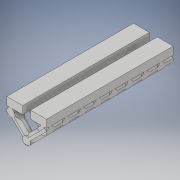
# Autodesk Inventor part: Basic_rail
Saved by Autodesk Inventor 2018.2 (Build 222227000, 227)
## iProperties
Created: 2018-04-02
Part Number: Basic_rail
Material: Generic
Document SubType Name: Modeling
Designer: martin
Density: 1 g/cm^3
Appearance: Default
Author: martin
Autodesk Inventor part; units mm, degrees
ref_plane "YZ Plane" through (0, 0, 0) normal (1, 0, 0) x (0, 1, 0)
ref_plane "XZ Plane" through (0, 0, 0) normal (0, 1, 0) x (-1, 0, 0)
ref_plane "XY Plane" through (0, 0, 0) normal (0, 0, 1) x (1, 0, 0)
sketch "Sketch1" plane through (0, 0, 0) normal (0, 0, 1) x (1, 0, 0)
  line L0 (0.0508, 0.0012) -> (1.1089, 0.0012)
  line L1 (1.1089, 0.0012) -> (2.1671, 1.0594)
  line L2 (2.1671, 1.0594) -> (2.1671, 2.1175)
  line L3 (2.1671, 2.1175) -> (1.1084, 3.1762)
  line L4 (1.1084, 3.1762) -> (0.0503, 3.1762)
  line L5 (0.0503, 3.1762) -> (-1.0079, 2.118)
  line L6 (-1.0079, 2.118) -> (-1.0079, 1.0599)
  line L7 (-1.0079, 1.0599) -> (0.0508, 0.0012)
  line L8 (6.4008, 0.0012) -> (7.4589, 0.0012)
  line L9 (7.4589, 0.0012) -> (8.5171, 1.0594)
  line L10 (8.5171, 1.0594) -> (8.5171, 2.1175)
  line L11 (8.5171, 2.1175) -> (7.4584, 3.1762)
  line L12 (7.4584, 3.1762) -> (6.4003, 3.1762)
  line L13 (6.4003, 3.1762) -> (5.3421, 2.118)
  line L14 (5.3421, 2.118) -> (5.3421, 1.0599)
  line L15 (5.3421, 1.0599) -> (6.4008, 0.0012)
  line L16 (0.0508, 0.0012) -> (1.1089, 0.0012)
  line L17 (1.1089, 0.0012) -> (2.1671, 1.0594)
  line L18 (2.1671, 1.0594) -> (2.1671, 2.1175)
  line L19 (2.1671, 2.1175) -> (1.1084, 3.1762)
  line L20 (1.1084, 3.1762) -> (0.0503, 3.1762)
  line L21 (0.0503, 3.1762) -> (-1.0079, 2.118)
  line L22 (-1.0079, 2.118) -> (-1.0079, 1.0599)
  line L23 (-1.0079, 1.0599) -> (0.0508, 0.0012)
  line L24 (12.7508, 0.0012) -> (13.8089, 0.0012)
  line L25 (13.8089, 0.0012) -> (14.8671, 1.0594)
  line L26 (14.8671, 1.0594) -> (14.8671, 2.1175)
  line L27 (14.8671, 2.1175) -> (13.8084, 3.1762)
  line L28 (13.8084, 3.1762) -> (12.7503, 3.1762)
  line L29 (12.7503, 3.1762) -> (11.6921, 2.118)
  line L30 (11.6921, 2.118) -> (11.6921, 1.0599)
  line L31 (11.6921, 1.0599) -> (12.7508, 0.0012)
  point P0 (0, 0)
  dimension "d0" = 0.0508
  dimension "d1" = 1.109
  dimension "d2" = 1.0582
  dimension "d3" = 135
  dimension "d4" = 135
  dimension "d5" = 135
  dimension "d6" = 3.175
  dimension "d8" = 1.0582
  dimension "d9" = 135
  dimension "d10" = 1.0582
  dimension "d11" = 1.0582
  dimension "d12" = 1.0582
  dimension "d13" = 135
  dimension "d14" = 135
  dimension "d15" = 135
  dimension "d16" = 3.175
  dimension "d17" = 3.175
  dimension "d18" = 1.0582
  dimension "d19" = 135
  dimension "d20" = 1.0582
  dimension "d21" = 1.0582
  dimension "d22" = 1.0582
  dimension "d23" = 135
  dimension "d24" = 135
  dimension "d25" = 135
  dimension "d26" = 3.175
  dimension "d27" = 3.175
  dimension "d28" = 1.0582
  dimension "d29" = 135
  dimension "d30" = 1.0582
  dimension "d31" = 1.0582
  dimension "d32" = 1.0582
  dimension "d33" = 135
  dimension "d34" = 135
  dimension "d35" = 135
  dimension "d36" = 3.175
  dimension "d37" = 3.175
  dimension "d38" = 1.0582
  dimension "d39" = 135
  dimension "d40" = 1.0582
  dimension "d41" = 1.0582
  dimension "d52" = 3.175
  dimension "d54" = 3.175
  constraints: 64 end point, 12 parallel, 4 horizontal, 4 perpendicular
  measures "d0" distance of point (0, 0) L0.start
  measures "d1" distance of L0.end point (0, 0)
  measures "d2" horizontal distance of L0.end L1.end
  measures "d3" angle of L0 L1
  measures "d4" angle of L2 L1
  measures "d5" angle of L3 L2
  measures "d6" distance between parallel lines of L0 L4
  measures "d8" distance of L0.start L0.end
  measures "d9" angle of L0 L7
  measures "d10" distance of L5.end L6.end
  measures "d11" distance of L3.end L4.end
  measures "d12" horizontal distance of L8.end L9.end
  measures "d13" angle of L8 L9
  measures "d14" angle of L10 L9
  measures "d15" angle of L11 L10
  measures "d16" distance between parallel lines of L8 L12
  measures "d17" distance between parallel lines of L14 L10
  measures "d18" distance of L8.start L8.end
  measures "d19" angle of L8 L15
  measures "d20" distance of L13.end L14.end
  measures "d21" distance of L11.end L12.end
  measures "d22" horizontal distance of L16.end L17.end
  measures "d23" angle of L16 L17
  measures "d24" angle of L18 L17
  measures "d25" angle of L19 L18
  measures "d26" distance between parallel lines of L16 L20
  measures "d27" distance between parallel lines of L22 L18
  measures "d28" distance of L16.start L16.end
  measures "d29" angle of L16 L23
  measures "d30" distance of L21.end L22.end
  measures "d31" distance of L19.end L20.end
  measures "d32" horizontal distance of L24.end L25.end
  measures "d33" angle of L24 L25
  measures "d34" angle of L26 L25
  measures "d35" angle of L27 L26
  measures "d36" distance between parallel lines of L24 L28
  measures "d37" distance between parallel lines of L30 L26
  measures "d38" distance of L24.start L24.end
  measures "d39" angle of L24 L31
  measures "d40" distance of L29.end L30.end
  measures "d41" distance of L27.end L28.end
  measures "d52" distance between parallel lines of L14 L18
  measures "d54" distance between parallel lines of L30 L10
extrude "Extrusion1" add sketch "Sketch1" along normal mid plane 50.8
sketch "Sketch2" plane through (14.8671, 1.0594, 25.4) normal (1, 0, 0) x (0, 0, -1)
  line L0 (1.0587, -1.0587) -> (2.1168, -1.0587)
  line L1 (2.1168, -1.0587) -> (3.175, -0.0005)
  line L2 (3.175, -0.0005) -> (3.175, 1.0577)
  line L3 (3.175, 1.0577) -> (2.1163, 2.1163)
  line L4 (2.1163, 2.1163) -> (1.0582, 2.1163)
  line L5 (1.0582, 2.1163) -> (0, 1.0582)
  line L6 (0, 1.0582) -> (0, 0)
  line L7 (0, 0) -> (1.0587, -1.0587)
  line L8 (7.4087, -1.0587) -> (8.4668, -1.0587)
  line L9 (8.4668, -1.0587) -> (9.525, -0.0005)
  line L10 (9.525, -0.0005) -> (9.525, 1.0577)
  line L11 (9.525, 1.0577) -> (8.4663, 2.1163)
  line L12 (8.4663, 2.1163) -> (7.4082, 2.1163)
  line L13 (7.4082, 2.1163) -> (6.35, 1.0582)
  line L14 (6.35, 1.0582) -> (6.35, 0)
  line L15 (6.35, 0) -> (7.4087, -1.0587)
  line L16 (1.0587, -1.0587) -> (2.1168, -1.0587)
  line L17 (2.1168, -1.0587) -> (3.175, -0.0005)
  line L18 (3.175, -0.0005) -> (3.175, 1.0577)
  line L19 (3.175, 1.0577) -> (2.1163, 2.1163)
  line L20 (2.1163, 2.1163) -> (1.0582, 2.1163)
  line L21 (1.0582, 2.1163) -> (0, 1.0582)
  line L22 (0, 1.0582) -> (0, 0)
  line L23 (0, 0) -> (1.0587, -1.0587)
  line L24 (13.7587, -1.0587) -> (14.8168, -1.0587)
  line L25 (14.8168, -1.0587) -> (15.875, -0.0005)
  line L26 (15.875, -0.0005) -> (15.875, 1.0577)
  line L27 (15.875, 1.0577) -> (14.8163, 2.1163)
  line L28 (14.8163, 2.1163) -> (13.7582, 2.1163)
  line L29 (13.7582, 2.1163) -> (12.7, 1.0582)
  line L30 (12.7, 1.0582) -> (12.7, 0)
  line L31 (12.7, 0) -> (13.7587, -1.0587)
  line L32 (21.1182, 2.1163) -> (20.06, 2.1163)
  line L33 (21.1663, 2.1163) -> (20.1082, 2.1163)
  line L34 (20.1082, 2.1163) -> (19.05, 1.0582)
  line L35 (20.06, 2.1163) -> (19.0018, 1.0582)
  line L36 (22.225, 1.0577) -> (21.1663, 2.1163)
  line L37 (22.1768, 1.0577) -> (21.1182, 2.1163)
  line L38 (19.05, 1.0582) -> (19.05, 0)
  line L39 (19.0018, 1.0582) -> (19.0018, 0)
  line L40 (22.225, -0.0005) -> (22.225, 1.0577)
  line L41 (22.1768, -0.0005) -> (22.1768, 1.0577)
  line L42 (20.1087, -1.0587) -> (21.1668, -1.0587)
  line L43 (20.0605, -1.0587) -> (21.1187, -1.0587)
  line L44 (19.0018, 0) -> (20.0605, -1.0587)
  line L45 (19.05, 0) -> (20.1087, -1.0587)
  line L46 (21.1187, -1.0587) -> (22.1768, -0.0005)
  line L47 (21.1668, -1.0587) -> (22.225, -0.0005)
  line L48 (31.7018, 1.0582) -> (31.7018, 0)
  line L49 (32.76, 2.1163) -> (31.7018, 1.0582)
  line L50 (31.7018, 0) -> (32.7605, -1.0587)
  line L51 (33.8182, 2.1163) -> (32.76, 2.1163)
  line L52 (32.7605, -1.0587) -> (33.8187, -1.0587)
  line L53 (33.8187, -1.0587) -> (34.8768, -0.0005)
  line L54 (34.8768, -0.0005) -> (34.8768, 1.0577)
  line L55 (34.8768, 1.0577) -> (33.8182, 2.1163)
  line L56 (25.3518, 1.0582) -> (25.3518, 0)
  line L57 (26.41, 2.1163) -> (25.3518, 1.0582)
  line L58 (25.3518, 0) -> (26.4105, -1.0587)
  line L59 (27.4682, 2.1163) -> (26.41, 2.1163)
  line L60 (26.4105, -1.0587) -> (27.4687, -1.0587)
  line L61 (27.4687, -1.0587) -> (28.5268, -0.0005)
  line L62 (28.5268, -0.0005) -> (28.5268, 1.0577)
  line L63 (28.5268, 1.0577) -> (27.4682, 2.1163)
  line L64 (38.0518, 1.0582) -> (38.0518, 0)
  line L65 (38.0518, 0) -> (39.1105, -1.0587)
  line L66 (39.11, 2.1163) -> (38.0518, 1.0582)
  line L67 (39.1105, -1.0587) -> (40.1687, -1.0587)
  line L68 (40.1682, 2.1163) -> (39.11, 2.1163)
  line L69 (40.1687, -1.0587) -> (41.2268, -0.0005)
  line L70 (41.2268, 1.0577) -> (40.1682, 2.1163)
  line L71 (41.2268, -0.0005) -> (41.2268, 1.0577)
  line L72 (44.4018, 1.0582) -> (44.4018, 0)
  line L73 (44.4018, 0) -> (45.4605, -1.0587)
  line L74 (45.46, 2.1163) -> (44.4018, 1.0582)
  line L75 (45.4605, -1.0587) -> (46.5187, -1.0587)
  line L76 (46.5182, 2.1163) -> (45.46, 2.1163)
  line L77 (46.5187, -1.0587) -> (47.5768, -0.0005)
  line L78 (47.5768, -0.0005) -> (47.5768, 1.0577)
  line L79 (47.5768, 1.0577) -> (46.5182, 2.1163)
  point P0 (25.4, -1.0594)
  point P1 (1.0079, -1.0599)
  point P2 (20.0579, -1.0599)
  dimension "d57" = 0.0508
  dimension "d58" = 1.109
  dimension "d59" = 1.0582
  dimension "d60" = 135
  dimension "d61" = 135
  dimension "d62" = 135
  dimension "d63" = 3.175
  dimension "d64" = 1.0582
  dimension "d65" = 135
  dimension "d66" = 1.0582
  dimension "d67" = 1.0582
  dimension "d68" = 1.0582
  dimension "d69" = 135
  dimension "d70" = 135
  dimension "d71" = 135
  dimension "d72" = 3.175
  dimension "d73" = 3.175
  dimension "d74" = 1.0582
  dimension "d75" = 135
  dimension "d76" = 1.0582
  dimension "d77" = 1.0582
  dimension "d78" = 1.0582
  dimension "d79" = 135
  dimension "d80" = 135
  dimension "d81" = 135
  dimension "d82" = 3.175
  dimension "d83" = 3.175
  dimension "d84" = 1.0582
  dimension "d85" = 135
  dimension "d86" = 1.0582
  dimension "d87" = 1.0582
  dimension "d88" = 1.0582
  dimension "d89" = 135
  dimension "d90" = 135
  dimension "d91" = 135
  dimension "d92" = 3.175
  dimension "d93" = 3.175
  dimension "d94" = 1.0582
  dimension "d95" = 135
  dimension "d96" = 1.0582
  dimension "d97" = 1.0582
  dimension "d98" = 3.175
  dimension "d99" = 3.175
  dimension "d100" = 0.0508
  dimension "d101" = 1.109
  dimension "d102" = 1.0582
  dimension "d103" = 135
  dimension "d104" = 135
  dimension "d105" = 135
  dimension "d106" = 3.175
  dimension "d107" = 1.0582
  dimension "d108" = 135
  dimension "d109" = 1.0582
  dimension "d110" = 1.0582
  dimension "d111" = 1.0582
  dimension "d112" = 135
  dimension "d113" = 135
  dimension "d114" = 135
  dimension "d115" = 3.175
  dimension "d116" = 3.175
  dimension "d117" = 1.0582
  dimension "d118" = 135
  dimension "d119" = 1.0582
  dimension "d120" = 1.0582
  constraints: 160 end point, 30 parallel, 10 horizontal, 10 perpendicular
  measures "d57" distance of point (1.008, -1.06) L0.start
  measures "d58" distance of L0.end point (1.008, -1.06)
  measures "d59" horizontal distance of L0.end L2.start
  measures "d60" angle of L0 L1
  measures "d61" angle of L2 L1
  measures "d62" angle of L3 L2
  measures "d63" distance between parallel lines of L0 L4
  measures "d64" distance of L0.start L0.end
  measures "d65" angle of L0 L7
  measures "d66" distance of L5.end L6.end
  measures "d67" distance of L4.start L4.end
  measures "d68" horizontal distance of L8.end L9.end
  measures "d69" angle of L8 L9
  measures "d70" angle of L10 L9
  measures "d71" angle of L11 L10
  measures "d72" distance between parallel lines of L8 L12
  measures "d73" distance between parallel lines of L14 L10
  measures "d74" distance of L15.end L8.end
  measures "d75" angle of L8 L15
  measures "d76" distance of L14.start L14.end
  measures "d77" distance of L12.start L13.start
  measures "d78" horizontal distance of L16.end L18.start
  measures "d79" angle of L16 L17
  measures "d80" angle of L18 L17
  measures "d81" angle of L19 L18
  measures "d82" distance between parallel lines of L16 L20
  measures "d83" distance between parallel lines of L22 L18
  measures "d84" distance of L16.start L16.end
  measures "d85" angle of L16 L23
  measures "d86" distance of L21.end L22.end
  measures "d87" distance of L20.start L20.end
  measures "d88" horizontal distance of L24.end L25.end
  measures "d89" angle of L24 L25
  measures "d90" angle of L26 L25
  measures "d91" angle of L27 L26
  measures "d92" distance between parallel lines of L24 L28
  measures "d93" distance between parallel lines of L30 L26
  measures "d94" distance of L31.end L24.end
  measures "d95" angle of L24 L31
  measures "d96" distance of L30.start L30.end
  measures "d97" distance of L28.start L29.start
  measures "d98" distance between parallel lines of L14 L18
  measures "d99" distance between parallel lines of L30 L10
  measures "d100" distance of point (20.058, -1.06) L45.end
  measures "d101" distance of L42.end point (20.058, -1.06)
  measures "d102" horizontal distance of L42.end L40.start
  measures "d103" angle of L42 L47
  measures "d104" angle of L40 L47
  measures "d105" angle of L36 L40
  measures "d106" distance between parallel lines of L42 L33
  measures "d107" distance of L45.end L42.end
  measures "d108" angle of L42 L45
  measures "d109" distance of L38.start L45.start
  measures "d110" distance of L33.start L33.end
  measures "d111" horizontal distance of L60.end L61.end
  measures "d112" angle of L60 L61
  measures "d113" angle of L62 L61
  measures "d114" angle of L63 L62
  measures "d115" distance between parallel lines of L60 L59
  measures "d116" distance between parallel lines of L56 L62
  measures "d117" distance of L58.end L60.end
  measures "d118" angle of L60 L58
  measures "d119" distance of L56.start L56.end
  measures "d120" distance of L59.start L57.start
extrude "Extrusion2" add sketch "Sketch2" against normal blind 15.875
sketch "Sketch5" plane through (13.8084, 3.1762, -25.4) normal (0.7071, 0.7071, 0) x (-0.7071, 0.7071, 0)
  line L0 (-1.5367, 3.1762) -> (-0.4786, 3.1762)
  line L1 (-0.4786, 3.1762) -> (0.5796, 4.2344)
  line L2 (0.5796, 4.2344) -> (0.5796, 5.2925)
  line L3 (0.5796, 5.2925) -> (-0.4791, 6.3512)
  line L4 (-0.4791, 6.3512) -> (-1.5372, 6.3512)
  line L5 (-1.5372, 6.3512) -> (-2.5954, 5.293)
  line L6 (-2.5954, 5.293) -> (-2.5954, 4.2349)
  line L7 (-2.5954, 4.2349) -> (-1.5367, 3.1762)
  line L8 (-1.5367, 3.1762) -> (-0.4786, 3.1762)
  line L9 (-0.4786, 3.1762) -> (0.5796, 4.2344)
  line L10 (0.5796, 4.2344) -> (0.5796, 5.2925)
  line L11 (0.5796, 5.2925) -> (-0.4791, 6.3512)
  line L12 (-0.4791, 6.3512) -> (-1.5372, 6.3512)
  line L13 (-1.5372, 6.3512) -> (-2.5954, 5.293)
  line L14 (-2.5954, 5.293) -> (-2.5954, 4.2349)
  line L15 (-2.5954, 4.2349) -> (-1.5367, 3.1762)
  line L16 (-0.4786, 9.5262) -> (0.5796, 10.5844)
  line L17 (0.5796, 10.5844) -> (0.5796, 11.6425)
  line L18 (0.5796, 10.5844) -> (0.5796, 11.6425)
  line L19 (-0.4786, 9.5262) -> (0.5796, 10.5844)
  line L20 (0.5796, 11.6425) -> (-0.4791, 12.7012)
  line L21 (0.5796, 11.6425) -> (-0.4791, 12.7012)
  line L22 (-1.5367, 9.5262) -> (-0.4786, 9.5262)
  line L23 (-1.5367, 9.5262) -> (-0.4786, 9.5262)
  line L24 (-0.4791, 12.7012) -> (-1.5372, 12.7012)
  line L25 (-0.4791, 12.7012) -> (-1.5372, 12.7012)
  line L26 (-1.5372, 12.7012) -> (-2.5954, 11.643)
  line L27 (-1.5372, 12.7012) -> (-2.5954, 11.643)
  line L28 (-2.5954, 11.643) -> (-2.5954, 10.5849)
  line L29 (-2.5954, 11.643) -> (-2.5954, 10.5849)
  line L30 (-2.5954, 10.5849) -> (-1.5367, 9.5262)
  line L31 (-2.5954, 10.5849) -> (-1.5367, 9.5262)
  line L32 (-0.4786, 15.8762) -> (0.5796, 16.9344)
  line L33 (0.5796, 16.9344) -> (0.5796, 17.9925)
  line L34 (0.5796, 16.9344) -> (0.5796, 17.9925)
  line L35 (-0.4786, 15.8762) -> (0.5796, 16.9344)
  line L36 (0.5796, 17.9925) -> (-0.4791, 19.0512)
  line L37 (0.5796, 17.9925) -> (-0.4791, 19.0512)
  line L38 (-1.5367, 15.8762) -> (-0.4786, 15.8762)
  line L39 (-1.5367, 15.8762) -> (-0.4786, 15.8762)
  line L40 (-0.4791, 19.0512) -> (-1.5372, 19.0512)
  line L41 (-0.4791, 19.0512) -> (-1.5372, 19.0512)
  line L42 (-1.5372, 19.0512) -> (-2.5954, 17.993)
  line L43 (-1.5372, 19.0512) -> (-2.5954, 17.993)
  line L44 (-2.5954, 17.993) -> (-2.5954, 16.9349)
  line L45 (-2.5954, 17.993) -> (-2.5954, 16.9349)
  line L46 (-2.5954, 16.9349) -> (-1.5367, 15.8762)
  line L47 (-2.5954, 16.9349) -> (-1.5367, 15.8762)
  line L48 (-0.4786, 22.2262) -> (0.5796, 23.2844)
  line L49 (0.5796, 23.2844) -> (0.5796, 24.3425)
  line L50 (0.5796, 23.2844) -> (0.5796, 24.3425)
  line L51 (-0.4786, 22.2262) -> (0.5796, 23.2844)
  line L52 (0.5796, 24.3425) -> (-0.4791, 25.4012)
  line L53 (0.5796, 24.3425) -> (-0.4791, 25.4012)
  line L54 (-1.5367, 22.2262) -> (-0.4786, 22.2262)
  line L55 (-1.5367, 22.2262) -> (-0.4786, 22.2262)
  line L56 (-0.4791, 25.4012) -> (-1.5372, 25.4012)
  line L57 (-0.4791, 25.4012) -> (-1.5372, 25.4012)
  line L58 (-1.5372, 25.4012) -> (-2.5954, 24.343)
  line L59 (-1.5372, 25.4012) -> (-2.5954, 24.343)
  line L60 (-2.5954, 24.343) -> (-2.5954, 23.2849)
  line L61 (-2.5954, 24.343) -> (-2.5954, 23.2849)
  line L62 (-2.5954, 23.2849) -> (-1.5367, 22.2262)
  line L63 (-2.5954, 23.2849) -> (-1.5367, 22.2262)
  line L64 (-0.4786, 28.5762) -> (0.5796, 29.6344)
  line L65 (0.5796, 29.6344) -> (0.5796, 30.6925)
  line L66 (0.5796, 29.6344) -> (0.5796, 30.6925)
  line L67 (-0.4786, 28.5762) -> (0.5796, 29.6344)
  line L68 (0.5796, 30.6925) -> (-0.4791, 31.7512)
  line L69 (0.5796, 30.6925) -> (-0.4791, 31.7512)
  line L70 (-1.5367, 28.5762) -> (-0.4786, 28.5762)
  line L71 (-1.5367, 28.5762) -> (-0.4786, 28.5762)
  line L72 (-0.4791, 31.7512) -> (-1.5372, 31.7512)
  line L73 (-0.4791, 31.7512) -> (-1.5372, 31.7512)
  line L74 (-1.5372, 31.7512) -> (-2.5954, 30.693)
  line L75 (-1.5372, 31.7512) -> (-2.5954, 30.693)
  line L76 (-2.5954, 30.693) -> (-2.5954, 29.6349)
  line L77 (-2.5954, 30.693) -> (-2.5954, 29.6349)
  line L78 (-2.5954, 29.6349) -> (-1.5367, 28.5762)
  line L79 (-2.5954, 29.6349) -> (-1.5367, 28.5762)
  line L80 (-0.4786, 34.9262) -> (0.5796, 35.9844)
  line L81 (0.5796, 35.9844) -> (0.5796, 37.0425)
  line L82 (0.5796, 35.9844) -> (0.5796, 37.0425)
  line L83 (-0.4786, 34.9262) -> (0.5796, 35.9844)
  line L84 (0.5796, 37.0425) -> (-0.4791, 38.1012)
  line L85 (0.5796, 37.0425) -> (-0.4791, 38.1012)
  line L86 (-1.5367, 34.9262) -> (-0.4786, 34.9262)
  line L87 (-1.5367, 34.9262) -> (-0.4786, 34.9262)
  line L88 (-0.4791, 38.1012) -> (-1.5372, 38.1012)
  line L89 (-0.4791, 38.1012) -> (-1.5372, 38.1012)
  line L90 (-1.5372, 38.1012) -> (-2.5954, 37.043)
  line L91 (-1.5372, 38.1012) -> (-2.5954, 37.043)
  line L92 (-2.5954, 37.043) -> (-2.5954, 35.9849)
  line L93 (-2.5954, 37.043) -> (-2.5954, 35.9849)
  line L94 (-2.5954, 35.9849) -> (-1.5367, 34.9262)
  line L95 (-2.5954, 35.9849) -> (-1.5367, 34.9262)
  line L96 (-0.4786, 47.6262) -> (0.5796, 48.6844)
  line L97 (0.5796, 48.6844) -> (0.5796, 49.7425)
  line L98 (0.5796, 48.6844) -> (0.5796, 49.7425)
  line L99 (-0.4786, 47.6262) -> (0.5796, 48.6844)
  line L100 (0.5796, 49.7425) -> (-0.4791, 50.8012)
  line L101 (0.5796, 49.7425) -> (-0.4791, 50.8012)
  line L102 (-1.5367, 47.6262) -> (-0.4786, 47.6262)
  line L103 (-1.5367, 47.6262) -> (-0.4786, 47.6262)
  line L104 (-0.4791, 50.8012) -> (-1.5372, 50.8012)
  line L105 (-0.4791, 50.8012) -> (-1.5372, 50.8012)
  line L106 (-1.5372, 50.8012) -> (-2.5954, 49.743)
  line L107 (-1.5372, 50.8012) -> (-2.5954, 49.743)
  line L108 (-2.5954, 49.743) -> (-2.5954, 48.6849)
  line L109 (-2.5954, 49.743) -> (-2.5954, 48.6849)
  line L110 (-2.5954, 48.6849) -> (-1.5367, 47.6262)
  line L111 (-2.5954, 48.6849) -> (-1.5367, 47.6262)
  line L112 (-2.5954, 43.393) -> (-2.5954, 42.3349)
  line L113 (-2.5954, 43.393) -> (-2.5954, 42.3349)
  line L114 (0.5796, 43.3925) -> (-0.4791, 44.4512)
  line L115 (0.5796, 43.3925) -> (-0.4791, 44.4512)
  line L116 (0.5796, 42.3344) -> (0.5796, 43.3925)
  line L117 (0.5796, 42.3344) -> (0.5796, 43.3925)
  line L118 (-1.5367, 41.2762) -> (-0.4786, 41.2762)
  line L119 (-1.5367, 41.2762) -> (-0.4786, 41.2762)
  line L120 (-0.4786, 41.2762) -> (0.5796, 42.3344)
  line L121 (-0.4786, 41.2762) -> (0.5796, 42.3344)
  line L122 (-0.4791, 44.4512) -> (-1.5372, 44.4512)
  line L123 (-0.4791, 44.4512) -> (-1.5372, 44.4512)
  line L124 (-1.5372, 44.4512) -> (-2.5954, 43.393)
  line L125 (-1.5372, 44.4512) -> (-2.5954, 43.393)
  line L126 (-2.5954, 42.3349) -> (-1.5367, 41.2762)
  line L127 (-2.5954, 42.3349) -> (-1.5367, 41.2762)
  point P0 (7.5181, 25.4)
  point P1 (-1.5875, 3.175)
  point P2 (-1.5875, 9.525)
  point P3 (-1.5875, 15.875)
  point P4 (-1.5875, 22.225)
  point P5 (-1.5875, 28.575)
  point P6 (-1.5875, 34.925)
  point P7 (-1.5875, 47.625)
  point P8 (-1.5875, 41.275)
  dimension "d342" = 0.0508
  dimension "d343" = 1.109
  dimension "d344" = 1.0582
  dimension "d345" = 135
  dimension "d346" = 135
  dimension "d347" = 135
  dimension "d348" = 3.175
  dimension "d349" = 1.0582
  dimension "d350" = 135
  dimension "d351" = 1.0582
  dimension "d352" = 1.0582
  dimension "d353" = 1.0582
  dimension "d354" = 135
  dimension "d355" = 135
  dimension "d356" = 135
  dimension "d357" = 3.175
  dimension "d358" = 3.175
  dimension "d359" = 1.0582
  dimension "d360" = 135
  dimension "d361" = 1.0582
  dimension "d362" = 1.0582
  dimension "d363" = 0.0508
  dimension "d364" = 1.109
  dimension "d365" = 1.0582
  dimension "d366" = 135
  dimension "d367" = 135
  dimension "d368" = 135
  dimension "d369" = 3.175
  dimension "d370" = 1.0582
  dimension "d371" = 135
  dimension "d372" = 1.0582
  dimension "d373" = 1.0582
  dimension "d374" = 1.0582
  dimension "d375" = 135
  dimension "d376" = 135
  dimension "d377" = 135
  dimension "d378" = 3.175
  dimension "d379" = 3.175
  dimension "d380" = 1.0582
  dimension "d381" = 135
  dimension "d382" = 1.0582
  dimension "d383" = 1.0582
  dimension "d384" = 0.0508
  dimension "d385" = 1.109
  dimension "d386" = 1.0582
  dimension "d387" = 135
  dimension "d388" = 135
  dimension "d389" = 135
  dimension "d390" = 3.175
  dimension "d391" = 1.0582
  dimension "d392" = 135
  dimension "d393" = 1.0582
  dimension "d394" = 1.0582
  dimension "d395" = 1.0582
  dimension "d396" = 135
  dimension "d397" = 135
  dimension "d398" = 135
  dimension "d399" = 3.175
  dimension "d400" = 3.175
  dimension "d401" = 1.0582
  dimension "d402" = 135
  dimension "d403" = 1.0582
  dimension "d404" = 1.0582
  dimension "d405" = 0.0508
  constraints: 256 end point, 48 parallel, 16 horizontal, 16 perpendicular
  measures "d342" distance of point (-1.587, 3.175) L0.start
  measures "d343" distance of L1.start point (-1.587, 3.175)
  measures "d344" horizontal distance of L1.start L1.end
  measures "d345" angle of L0 L1
  measures "d346" angle of L2 L1
  measures "d347" angle of L3 L2
  measures "d348" distance between parallel lines of L0 L4
  measures "d349" distance of L0.start L1.start
  measures "d350" angle of L0 L7
  measures "d351" distance of L5.end L6.end
  measures "d352" distance of L3.end L4.end
  measures "d353" horizontal distance of L9.start L10.start
  measures "d354" angle of L8 L9
  measures "d355" angle of L10 L9
  measures "d356" angle of L11 L10
  measures "d357" distance between parallel lines of L8 L12
  measures "d358" distance between parallel lines of L14 L10
  measures "d359" distance of L8.start L9.start
  measures "d360" angle of L8 L15
  measures "d361" distance of L13.end L14.end
  measures "d362" distance of L11.end L12.end
  measures "d363" distance of point (-1.587, 9.525) L22.start
  measures "d364" distance of L22.end point (-1.587, 9.525)
  measures "d365" horizontal distance of L22.end L17.start
  measures "d366" angle of L22 L16
  measures "d367" angle of L17 L16
  measures "d368" angle of L20 L17
  measures "d369" distance between parallel lines of L22 L24
  measures "d370" distance of L22.start L22.end
  measures "d371" angle of L22 L30
  measures "d372" distance of L28.start L28.end
  measures "d373" distance of L20.end L24.end
  measures "d374" horizontal distance of L23.end L18.start
  measures "d375" angle of L23 L19
  measures "d376" angle of L18 L19
  measures "d377" angle of L21 L18
  measures "d378" distance between parallel lines of L23 L25
  measures "d379" distance between parallel lines of L29 L18
  measures "d380" distance of L23.start L23.end
  measures "d381" angle of L23 L31
  measures "d382" distance of L29.start L29.end
  measures "d383" distance of L21.end L25.end
  measures "d384" distance of point (-1.587, 15.875) L38.start
  measures "d385" distance of L38.end point (-1.587, 15.875)
  measures "d386" horizontal distance of L38.end L33.start
  measures "d387" angle of L38 L32
  measures "d388" angle of L33 L32
  measures "d389" angle of L36 L33
  measures "d390" distance between parallel lines of L38 L40
  measures "d391" distance of L38.start L38.end
  measures "d392" angle of L38 L46
  measures "d393" distance of L44.start L44.end
  measures "d394" distance of L36.end L40.end
  measures "d395" horizontal distance of L39.end L34.start
  measures "d396" angle of L39 L35
  measures "d397" angle of L34 L35
  measures "d398" angle of L37 L34
  measures "d399" distance between parallel lines of L39 L41
  measures "d400" distance between parallel lines of L45 L34
  measures "d401" distance of L39.start L39.end
  measures "d402" angle of L39 L47
  measures "d403" distance of L45.start L45.end
  measures "d404" distance of L37.end L41.end
  measures "d405" distance of point (-1.587, 22.225) L54.start
extrude "Extrusion3" add sketch "Sketch5" against normal blind 12.7
sketch "Sketch7" plane through (0.0503, 3.1762, -25.4) normal (-0.7071, 0.7071, 0) x (-0.7071, -0.7071, 0)
  line L0 (1.5875, 3.175) -> (2.6457, 4.2332)
  line L1 (2.6457, 4.2332) -> (2.6457, 5.2913)
  line L2 (2.6457, 4.2332) -> (2.6457, 5.2913)
  line L3 (1.5875, 3.175) -> (2.6457, 4.2332)
  line L4 (2.6457, 5.2913) -> (1.587, 6.35)
  line L5 (2.6457, 5.2913) -> (1.587, 6.35)
  line L6 (0.5293, 3.175) -> (1.5875, 3.175)
  line L7 (0.5293, 3.175) -> (1.5875, 3.175)
  line L8 (1.587, 6.35) -> (0.5288, 6.35)
  line L9 (1.587, 6.35) -> (0.5288, 6.35)
  line L10 (0.5288, 6.35) -> (-0.5293, 5.2918)
  line L11 (0.5288, 6.35) -> (-0.5293, 5.2918)
  line L12 (-0.5293, 5.2918) -> (-0.5293, 4.2337)
  line L13 (-0.5293, 5.2918) -> (-0.5293, 4.2337)
  line L14 (-0.5293, 4.2337) -> (0.5293, 3.175)
  line L15 (-0.5293, 4.2337) -> (0.5293, 3.175)
  line L16 (-0.5293, 11.6418) -> (-0.5293, 10.5837)
  line L17 (-0.5293, 11.6418) -> (-0.5293, 10.5837)
  line L18 (2.6457, 11.6413) -> (1.587, 12.7)
  line L19 (2.6457, 11.6413) -> (1.587, 12.7)
  line L20 (2.6457, 10.5832) -> (2.6457, 11.6413)
  line L21 (2.6457, 10.5832) -> (2.6457, 11.6413)
  line L22 (0.5293, 9.525) -> (1.5875, 9.525)
  line L23 (0.5293, 9.525) -> (1.5875, 9.525)
  line L24 (1.5875, 9.525) -> (2.6457, 10.5832)
  line L25 (1.5875, 9.525) -> (2.6457, 10.5832)
  line L26 (1.587, 12.7) -> (0.5288, 12.7)
  line L27 (1.587, 12.7) -> (0.5288, 12.7)
  line L28 (0.5288, 12.7) -> (-0.5293, 11.6418)
  line L29 (0.5288, 12.7) -> (-0.5293, 11.6418)
  line L30 (-0.5293, 10.5837) -> (0.5293, 9.525)
  line L31 (-0.5293, 10.5837) -> (0.5293, 9.525)
  line L32 (-0.5293, 17.9918) -> (-0.5293, 16.9337)
  line L33 (-0.5293, 17.9918) -> (-0.5293, 16.9337)
  line L34 (2.6457, 17.9913) -> (1.587, 19.05)
  line L35 (2.6457, 17.9913) -> (1.587, 19.05)
  line L36 (2.6457, 16.9332) -> (2.6457, 17.9913)
  line L37 (2.6457, 16.9332) -> (2.6457, 17.9913)
  line L38 (0.5293, 15.875) -> (1.5875, 15.875)
  line L39 (0.5293, 15.875) -> (1.5875, 15.875)
  line L40 (1.5875, 15.875) -> (2.6457, 16.9332)
  line L41 (1.5875, 15.875) -> (2.6457, 16.9332)
  line L42 (1.587, 19.05) -> (0.5288, 19.05)
  line L43 (1.587, 19.05) -> (0.5288, 19.05)
  line L44 (0.5288, 19.05) -> (-0.5293, 17.9918)
  line L45 (0.5288, 19.05) -> (-0.5293, 17.9918)
  line L46 (-0.5293, 16.9337) -> (0.5293, 15.875)
  line L47 (-0.5293, 16.9337) -> (0.5293, 15.875)
  line L48 (-0.5293, 24.3418) -> (-0.5293, 23.2837)
  line L49 (-0.5293, 24.3418) -> (-0.5293, 23.2837)
  line L50 (2.6457, 24.3413) -> (1.587, 25.4)
  line L51 (2.6457, 24.3413) -> (1.587, 25.4)
  line L52 (2.6457, 23.2832) -> (2.6457, 24.3413)
  line L53 (2.6457, 23.2832) -> (2.6457, 24.3413)
  line L54 (0.5293, 22.225) -> (1.5875, 22.225)
  line L55 (0.5293, 22.225) -> (1.5875, 22.225)
  line L56 (1.5875, 22.225) -> (2.6457, 23.2832)
  line L57 (1.5875, 22.225) -> (2.6457, 23.2832)
  line L58 (1.587, 25.4) -> (0.5288, 25.4)
  line L59 (1.587, 25.4) -> (0.5288, 25.4)
  line L60 (0.5288, 25.4) -> (-0.5293, 24.3418)
  line L61 (0.5288, 25.4) -> (-0.5293, 24.3418)
  line L62 (-0.5293, 23.2837) -> (0.5293, 22.225)
  line L63 (-0.5293, 23.2837) -> (0.5293, 22.225)
  line L64 (-0.5293, 30.6918) -> (-0.5293, 29.6337)
  line L65 (-0.5293, 30.6918) -> (-0.5293, 29.6337)
  line L66 (2.6457, 30.6913) -> (1.587, 31.75)
  line L67 (2.6457, 30.6913) -> (1.587, 31.75)
  line L68 (2.6457, 29.6332) -> (2.6457, 30.6913)
  line L69 (2.6457, 29.6332) -> (2.6457, 30.6913)
  line L70 (0.5293, 28.575) -> (1.5875, 28.575)
  line L71 (0.5293, 28.575) -> (1.5875, 28.575)
  line L72 (1.5875, 28.575) -> (2.6457, 29.6332)
  line L73 (1.5875, 28.575) -> (2.6457, 29.6332)
  line L74 (1.587, 31.75) -> (0.5288, 31.75)
  line L75 (1.587, 31.75) -> (0.5288, 31.75)
  line L76 (0.5288, 31.75) -> (-0.5293, 30.6918)
  line L77 (0.5288, 31.75) -> (-0.5293, 30.6918)
  line L78 (-0.5293, 29.6337) -> (0.5293, 28.575)
  line L79 (-0.5293, 29.6337) -> (0.5293, 28.575)
  line L80 (-0.5293, 37.0418) -> (-0.5293, 35.9837)
  line L81 (-0.5293, 37.0418) -> (-0.5293, 35.9837)
  line L82 (2.6457, 37.0413) -> (1.587, 38.1)
  line L83 (2.6457, 37.0413) -> (1.587, 38.1)
  line L84 (2.6457, 35.9832) -> (2.6457, 37.0413)
  line L85 (2.6457, 35.9832) -> (2.6457, 37.0413)
  line L86 (0.5293, 34.925) -> (1.5875, 34.925)
  line L87 (0.5293, 34.925) -> (1.5875, 34.925)
  line L88 (1.5875, 34.925) -> (2.6457, 35.9832)
  line L89 (1.5875, 34.925) -> (2.6457, 35.9832)
  line L90 (1.587, 38.1) -> (0.5288, 38.1)
  line L91 (1.587, 38.1) -> (0.5288, 38.1)
  line L92 (0.5288, 38.1) -> (-0.5293, 37.0418)
  line L93 (0.5288, 38.1) -> (-0.5293, 37.0418)
  line L94 (-0.5293, 35.9837) -> (0.5293, 34.925)
  line L95 (-0.5293, 35.9837) -> (0.5293, 34.925)
  line L96 (-0.5293, 49.7418) -> (-0.5293, 48.6837)
  line L97 (-0.5293, 49.7418) -> (-0.5293, 48.6837)
  line L98 (2.6457, 49.7413) -> (1.587, 50.8)
  line L99 (2.6457, 49.7413) -> (1.587, 50.8)
  line L100 (2.6457, 48.6832) -> (2.6457, 49.7413)
  line L101 (2.6457, 48.6832) -> (2.6457, 49.7413)
  line L102 (0.5293, 47.625) -> (1.5875, 47.625)
  line L103 (0.5293, 47.625) -> (1.5875, 47.625)
  line L104 (1.5875, 47.625) -> (2.6457, 48.6832)
  line L105 (1.5875, 47.625) -> (2.6457, 48.6832)
  line L106 (1.587, 50.8) -> (0.5288, 50.8)
  line L107 (1.587, 50.8) -> (0.5288, 50.8)
  line L108 (0.5288, 50.8) -> (-0.5293, 49.7418)
  line L109 (0.5288, 50.8) -> (-0.5293, 49.7418)
  line L110 (-0.5293, 48.6837) -> (0.5293, 47.625)
  line L111 (-0.5293, 48.6837) -> (0.5293, 47.625)
  line L112 (2.6457, 43.3913) -> (1.587, 44.45)
  line L113 (1.587, 44.45) -> (0.5288, 44.45)
  line L114 (1.587, 44.45) -> (0.5288, 44.45)
  line L115 (0.5288, 44.45) -> (-0.5293, 43.3918)
  line L116 (0.5288, 44.45) -> (-0.5293, 43.3918)
  line L117 (2.6457, 43.3913) -> (1.587, 44.45)
  line L118 (2.6457, 42.3332) -> (2.6457, 43.3913)
  line L119 (2.6457, 42.3332) -> (2.6457, 43.3913)
  line L120 (1.5875, 41.275) -> (2.6457, 42.3332)
  line L121 (1.5875, 41.275) -> (2.6457, 42.3332)
  line L122 (-0.5293, 43.3918) -> (-0.5293, 42.3337)
  line L123 (-0.5293, 43.3918) -> (-0.5293, 42.3337)
  line L124 (0.5293, 41.275) -> (1.5875, 41.275)
  line L125 (-0.5293, 42.3337) -> (0.5293, 41.275)
  line L126 (-0.5293, 42.3337) -> (0.5293, 41.275)
  line L127 (0.5293, 41.275) -> (1.5875, 41.275)
  point P0 (2.2815, 25.4)
  point P1 (0.4786, 3.1738)
  point P2 (0.4786, 9.5238)
  point P3 (0.4786, 15.8738)
  point P4 (0.4786, 22.2238)
  point P5 (0.4786, 28.5738)
  point P6 (0.4786, 34.9238)
  point P7 (0.4786, 47.6238)
  point P8 (0.4786, 41.2738)
  dimension "d514" = 0.0508
  dimension "d515" = 1.109
  dimension "d516" = 1.0582
  dimension "d517" = 135
  dimension "d518" = 135
  dimension "d519" = 135
  dimension "d520" = 3.175
  dimension "d521" = 1.0582
  dimension "d522" = 135
  dimension "d523" = 1.0582
  dimension "d524" = 1.0582
  dimension "d525" = 1.0582
  dimension "d526" = 135
  dimension "d527" = 135
  dimension "d528" = 135
  dimension "d529" = 3.175
  dimension "d530" = 3.175
  dimension "d531" = 1.0582
  dimension "d532" = 135
  dimension "d533" = 1.0582
  dimension "d534" = 1.0582
  dimension "d535" = 0.0508
  dimension "d536" = 1.109
  dimension "d537" = 1.0582
  dimension "d538" = 135
  dimension "d539" = 135
  dimension "d540" = 135
  dimension "d541" = 3.175
  dimension "d542" = 1.0582
  dimension "d543" = 135
  dimension "d544" = 1.0582
  dimension "d545" = 1.0582
  dimension "d546" = 1.0582
  dimension "d547" = 135
  dimension "d548" = 135
  dimension "d549" = 135
  dimension "d550" = 3.175
  dimension "d551" = 3.175
  dimension "d552" = 1.0582
  dimension "d553" = 135
  dimension "d554" = 1.0582
  dimension "d555" = 1.0582
  dimension "d556" = 0.0508
  dimension "d557" = 1.109
  dimension "d558" = 1.0582
  dimension "d559" = 135
  dimension "d560" = 135
  dimension "d561" = 135
  dimension "d562" = 3.175
  dimension "d563" = 1.0582
  dimension "d564" = 135
  dimension "d565" = 1.0582
  dimension "d566" = 1.0582
  dimension "d567" = 1.0582
  dimension "d568" = 135
  dimension "d569" = 135
  dimension "d570" = 135
  dimension "d571" = 3.175
  dimension "d572" = 3.175
  dimension "d573" = 1.0582
  dimension "d574" = 135
  dimension "d575" = 1.0582
  dimension "d576" = 1.0582
  dimension "d577" = 0.0508
  constraints: 256 end point, 48 parallel, 16 horizontal, 16 perpendicular
  measures "d514" distance of point (0.479, 3.174) L6.start
  measures "d515" distance of L6.end point (0.479, 3.174)
  measures "d516" horizontal distance of L6.end L1.start
  measures "d517" angle of L6 L0
  measures "d518" angle of L1 L0
  measures "d519" angle of L4 L1
  measures "d520" distance between parallel lines of L6 L8
  measures "d521" distance of L6.start L6.end
  measures "d522" angle of L6 L14
  measures "d523" distance of L12.start L12.end
  measures "d524" distance of L8.start L10.start
  measures "d525" horizontal distance of L7.end L2.start
  measures "d526" angle of L7 L3
  measures "d527" angle of L2 L3
  measures "d528" angle of L5 L2
  measures "d529" distance between parallel lines of L7 L9
  measures "d530" distance between parallel lines of L13 L2
  measures "d531" distance of L15.end L7.end
  measures "d532" angle of L7 L15
  measures "d533" distance of L13.start L13.end
  measures "d534" distance of L9.start L11.start
  measures "d535" distance of point (0.479, 9.524) L22.start
  measures "d536" distance of L22.end point (0.479, 9.524)
  measures "d537" horizontal distance of L22.end L24.end
  measures "d538" angle of L22 L24
  measures "d539" angle of L20 L24
  measures "d540" angle of L19 L20
  measures "d541" distance between parallel lines of L22 L26
  measures "d542" distance of L22.start L22.end
  measures "d543" angle of L22 L30
  measures "d544" distance of L17.start L30.start
  measures "d545" distance of L19.end L26.end
  measures "d546" horizontal distance of L23.end L25.end
  measures "d547" angle of L23 L25
  measures "d548" angle of L21 L25
  measures "d549" angle of L18 L21
  measures "d550" distance between parallel lines of L23 L27
  measures "d551" distance between parallel lines of L16 L21
  measures "d552" distance of L23.start L23.end
  measures "d553" angle of L23 L31
  measures "d554" distance of L16.start L31.start
  measures "d555" distance of L18.end L27.end
  measures "d556" distance of point (0.479, 15.874) L38.start
  measures "d557" distance of L38.end point (0.479, 15.874)
  measures "d558" horizontal distance of L38.end L40.end
  measures "d559" angle of L38 L40
  measures "d560" angle of L36 L40
  measures "d561" angle of L35 L36
  measures "d562" distance between parallel lines of L38 L42
  measures "d563" distance of L38.start L38.end
  measures "d564" angle of L38 L46
  measures "d565" distance of L33.start L46.start
  measures "d566" distance of L35.end L42.end
  measures "d567" horizontal distance of L39.end L41.end
  measures "d568" angle of L39 L41
  measures "d569" angle of L37 L41
  measures "d570" angle of L34 L37
  measures "d571" distance between parallel lines of L39 L43
  measures "d572" distance between parallel lines of L32 L37
  measures "d573" distance of L39.start L39.end
  measures "d574" angle of L39 L47
  measures "d575" distance of L32.start L47.start
  measures "d576" distance of L34.end L43.end
  measures "d577" distance of point (0.479, 22.224) L54.start
extrude "Extrusion4" add sketch "Sketch7" against normal blind 12.7
sketch "Sketch8" plane through (14.8954, 2.0892, 25.4012) normal (0, 0, 1) x (0.7071, 0.7071, 0)
  line L0 (-11.31, -1.0415) -> (-10.2518, -1.0415)
  line L1 (-10.2518, -1.0415) -> (-9.1936, 0.0166)
  line L2 (-9.1936, 0.0166) -> (-9.1936, 1.0748)
  line L3 (-9.1936, 1.0748) -> (-10.2523, 2.1335)
  line L4 (-10.2523, 2.1335) -> (-11.3105, 2.1335)
  line L5 (-11.3105, 2.1335) -> (-12.3686, 1.0753)
  line L6 (-12.3686, 1.0753) -> (-12.3686, 0.0171)
  line L7 (-12.3686, 0.0171) -> (-11.31, -1.0415)
  point P0 (-12.01, 9.0554)
  dimension "d728" = 1.0582
  dimension "d729" = 135
  dimension "d730" = 135
  dimension "d731" = 135
  dimension "d732" = 3.175
  dimension "d733" = 3.175
  dimension "d734" = 1.0582
  dimension "d735" = 135
  dimension "d736" = 1.0582
  dimension "d737" = 1.0582
  constraints: 16 end point, 3 parallel, 1 horizontal, 1 perpendicular
  measures "d728" horizontal distance of L0.end L2.start
  measures "d729" angle of L0 L1
  measures "d730" angle of L2 L1
  measures "d731" angle of L3 L2
  measures "d732" distance between parallel lines of L0 L4
  measures "d733" distance between parallel lines of L6 L2
  measures "d734" distance of L7.end L0.end
  measures "d735" angle of L0 L7
  measures "d736" distance of L6.start L6.end
  measures "d737" distance of L4.start L5.start
extrude "Extrusion5" add sketch "Sketch8" against normal blind 50.8
sketch "Sketch10" plane through (0, 0, 25.4) normal (0, 0, 1) x (1, 0, 0)
  line L0 (9.8132, 0.0007) -> (6.8938, -2.9187) projected
  line L1 (6.8938, -2.9187) -> (11.5339, 1.7213)
  line L2 (14.1472, 2.8375) -> (7.6463, -3.6634) projected
  line L3 (11.5339, 1.7213) -> (11.5339, 4.3944)
  line L4 (12.7498, 3.1757) -> (7.4589, 3.1757) projected
  line L5 (11.5339, 4.3944) -> (2.0089, 4.3944)
  line L6 (2.0089, 4.3944) -> (2.0089, 1.9662)
  line L7 (2.0089, 1.9662) -> (6.8938, -2.9187)
  point P0 (0, 0)
  dimension "d745" = 9.525
  constraints: 10 end point, 4 perpendicular, 1 parallel
  measures "d745" distance between parallel lines of L6 L3
extrude "Extrusion6" cut sketch "Sketch10" against normal through all
sketch "Sketch11" plane through (0, 0, 25.4) normal (0, 0, 1) x (1, 0, 0)
  line L0 (0.0498, 3.1757) -> (-1.0079, 3.1757) projected
  line L1 (-1.0079, 6.3507) -> (5.3421, 6.3507)
  line L2 (5.3421, 6.3507) -> (5.3421, 3.1757)
  line L3 (5.3421, 3.1757) -> (-1.0079, 3.1757)
  line L4 (-1.0079, 3.1757) -> (-1.0079, 6.3507)
  line L5 (8.5171, 6.3507) -> (14.8671, 6.3507)
  line L6 (14.8671, 6.3507) -> (14.8671, 3.1757)
  line L7 (14.8671, 3.1757) -> (8.5171, 3.1757)
  line L8 (8.5171, 3.1757) -> (8.5171, 6.3507)
  point P0 (0, 0)
  dimension "d748" = 6.35
  dimension "d749" = 3.175
  dimension "d750" = 6.35
  dimension "d751" = 3.175
  dimension "d752" = 3.175
  constraints: 16 end point, 4 parallel, 2 horizontal, 2 perpendicular
  measures "d748" distance of L2.end L3.end
  measures "d749" distance of L1.end L2.end
  measures "d750" distance of L6.end L7.end
  measures "d751" distance of L5.end L6.end
  measures "d752" distance between parallel lines of L8 L2
extrude "Extrusion7" add sketch "Sketch11" against normal blind 50.8
sketch "Sketch12" plane through (0, 0, 25.4) normal (0, 0, 1) x (1, 0, 0)
  line L0 (14.8671, 6.3507) -> (14.8671, 3.1757) projected
  line L1 (14.8671, 6.3507) -> (15.875, 6.3507)
  line L2 (15.875, 6.3507) -> (15.875, -1.5875)
  line L3 (15.875, -1.5875) -> (14.8671, -1.5875)
  line L4 (14.8671, -1.5875) -> (14.8671, 6.3507)
  line L5 (-1.0079, 3.1757) -> (-1.0079, 6.3507) projected
  line L6 (-1.0079, 6.3507) -> (-3.175, 6.3507)
  line L7 (-3.175, 6.3507) -> (-3.175, -1.5875)
  line L8 (-3.175, -1.5875) -> (-1.0079, -1.5875)
  line L9 (-1.0079, -1.5875) -> (-1.0079, 6.3507)
  line L10 (4.4414, -6.5169) -> (9.525, -6.5169)
  line L11 (9.525, -6.5169) -> (9.525, -8.5429)
  line L12 (9.525, -8.5429) -> (4.4414, -8.5429)
  line L13 (4.4414, -8.5429) -> (4.4414, -6.5169)
  point P0 (0, 0)
  constraints: 24 end point, 6 parallel, 3 horizontal, 3 perpendicular
extrude "Extrusion8" cut sketch "Sketch12" against normal blind 50.8
sketch "Sketch13" plane through (6.1374, -3.6517, 25.4012) normal (0, 0, 1) x (1, 0, 0)
  line L0 (1.4972, -2.9929) -> (0.0242, -2.9929) projected
  line L1 (1.4972, -2.9929) -> (9.4166, 4.9265)
  line L2 (7.9746, 3.9559) -> (8.7297, 4.711) projected
  line L3 (9.4166, 4.9265) -> (9.4166, -2.9929)
  line L4 (9.4166, -2.9929) -> (1.4972, -2.9929)
  line L5 (0.0242, -2.9929) -> (-7.835, 4.8663)
  line L6 (-7.835, 4.8663) -> (-8.1831, -2.7575)
  line L7 (-8.1831, -2.7575) -> (0.0177, -3.4857)
  line L8 (0.0177, -3.4857) -> (0.0242, -2.9929)
  line L9 (0.0242, -2.9929) -> (-0.2222, -3.2394) projected
  point P0 (-6.1374, 3.6517)
  dimension "d757" = 90
  constraints: 14 end point, 3 point on line, 1 parallel, 1 perpendicular
  measures "d757" angle of L1 L5
extrude "Extrusion9" cut sketch "Sketch13" against normal blind 50.8 contours L8 L7 L6 L5
sketch "Sketch14" plane through (6.1374, -3.6517, 25.4012) normal (0, 0, 1) x (1, 0, 0)
  line L0 (1.2521, -3.175) -> (10.7771, 6.35)
  line L1 (10.7771, 6.35) -> (10.7771, -3.175)
  line L2 (10.7771, -3.175) -> (1.484, -2.9431)
  point P0 (-6.1374, 3.6517)
  constraints: 6 end point, 1 point on line
extrude "Extrusion10" cut sketch "Sketch14" against normal blind 50.8
sketch "Sketch15" plane through (0, 0, 25.4) normal (0, 0, 1) x (1, 0, 0)
  point P0 (0, 0)
body "Solid1"
